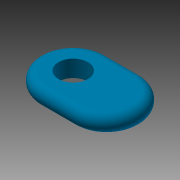
# Autodesk Inventor part: Plectrum
Saved by Autodesk Inventor 2014 SP1 (Build 180222100, 222)
## iProperties
Created: 2016-12-01
Part Number: Plectrum
Material: Generic
Document SubType Name: Modeling
Designer: danielsikar
Density: 1 g/cm^3
Appearance: Sky Blue Medium
Author: danielsikar
Autodesk Inventor part; units mm, degrees
ref_plane "YZ Plane" through (0, 0, 0) normal (1, 0, 0) x (0, 1, 0)
ref_plane "XZ Plane" through (0, 0, 0) normal (0, 1, 0) x (-1, 0, 0)
ref_plane "XY Plane" through (0, 0, 0) normal (0, 0, 1) x (1, 0, 0)
sketch "Sketch3" plane through (0, 0, 0) normal (0, 0, 1) x (1, 0, 0)
  line L0 (0, 0) -> (12, 0)
  line L1 (12, 0) -> (12, 8)
  line L2 (12, 8) -> (0, 8)
  line L3 (0, 8) -> (0, 0)
  dimension "d6" = 12
  dimension "d7" = 8
  constraints: 8 end point, 2 parallel, 1 horizontal, 1 perpendicular
  measures "d6" distance of L2.end L1.end
  measures "d7" distance of L1.end L0.end
extrude "Extrusion2" add sketch "Sketch3" along normal blind 2
fillet "Fillet2" radius 4 4 edges at (0, 8, 1) (0, 0, 1) (12, 0, 1) (12, 8, 1)
sketch "Sketch4" plane through (0, 0, 2) normal (0, 0, 1) x (1, 0, 0)
  arc A0 (4, 8) -> (4, 0) centre (4, 4) ccw projected
  circle A1 centre (4, 4) radius 1.75
  point P0 (0, 0)
  dimension "d11" = 3.5
  constraints: 1 centre point, 1 coincident
  measures "d11" diameter of A1
extrude "Extrusion3" cut sketch "Sketch4" against normal blind 2
fillet "Fillet3" radius 1 8 edges at (1.1714, 6.8286, 2) (6, 0, 2) (10.8286, 1.1714, 2) (6, 8, 2) (1.1714, 6.8286, 0) (6, 0, 0) (10.8286, 1.1714, 0) (6, 8, 0)
body "Solid2"
